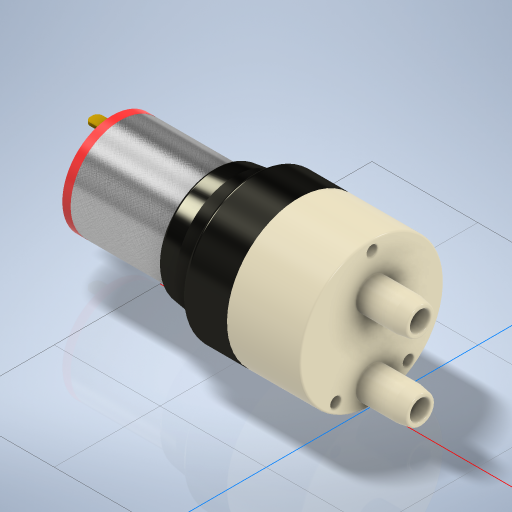
# Autodesk Inventor part: pump
Saved by Autodesk Inventor 2024 (Build 280153000, 153)
## iProperties
Created: 2023-05-18
Part Number: pump
Material: Generic
Document SubType Name: Modeling
Designer: jeff7
Density: 1 g/cm^3
Appearance: Default
Author: jeff7
Autodesk Inventor part; units mm, degrees
sketch "Sketch1" plane through (0, 0, 0) normal (1, 0, 0) x (0, 1, 0)
  circle A0 centre (0, 0) radius 17.25
  dimension "d0" = 34.5
  constraints: 2 coincident, 1 centre point
  measures "d0" diameter of A0
extrude "Extrusion1" add sketch "Sketch1" against normal blind 28.4
sketch "Sketch2" plane through (-28.4, 0, 0) normal (-1, 0, 0) x (0, 0, 1)
  circle A0 centre (0, 0) radius 14.1
  dimension "d3" = 28.2
  constraints: 1 centre point, 1 coincident
  measures "d3" diameter of A0
extrude "Extrusion2" add sketch "Sketch2" along normal blind 9.5
sketch "Sketch3" plane through (-37.9, 0, 0) normal (-1, 0, 0) x (0, 0, 1)
  circle A0 centre (0, 0) radius 17.25 projected
  circle A1 centre (0, 0) radius 11.95
  dimension "d6" = 23.9
  constraints: 1 centre point, 1 coincident
  measures "d6" diameter of A1
extrude "Extrusion3" add sketch "Sketch3" along normal blind 24.4 contours A1
sketch "Sketch5" plane through (0, 0, 0) normal (1, 0, 0) x (0, 0, -1)
  circle A0 centre (0, -12.35) radius 3.85
  circle A1 centre (0, 6.1) radius 3.85
  circle A2 centre (0, -12.35) radius 2.35
  circle A3 centre (0, 6.1) radius 2.35
  circle A4 centre (0, 0) radius 17.25 projected
  dimension "d9" = 7.7
  dimension "d10" = 7.7
  dimension "d11" = 4.7
  dimension "d12" = 4.7
  dimension "d13" = 1.05
  dimension "d14" = 15
  constraints: 4 centre point, 2 coincident, 2 vertical alignment
  measures "d9" diameter of A0
  measures "d10" diameter of A1
  measures "d11" diameter of A2
  measures "d12" diameter of A3
extrude "Extrusion4" add sketch "Sketch5" along normal blind 11.7 contours A0 | A1
sketch "Sketch6" plane through (0, 0, 0) normal (1, 0, 0) x (0, 0, -1)
  circle A0 centre (0, 14.95) radius 1.3
  circle A1 centre (8.7, -12.1578) radius 1.3
  circle A2 centre (-8.7, -12.1578) radius 1.3
  circle A3 centre (0, 0) radius 17.25 projected
  dimension "d17" = 2.6
  dimension "d18" = 2.6
  dimension "d19" = 2.6
  dimension "d20" = 1
  dimension "d21" = 17.4
  dimension "d22" = 1
  dimension "d23" = 1
  constraints: 3 centre point, 1 horizontal alignment, 1 vertical alignment
  measures "d17" diameter of A0
  measures "d18" diameter of A2
  measures "d19" diameter of A1
  measures "d21" distance of A1.centre A2.centre
extrude "Extrusion5" cut sketch "Sketch6" against normal blind 10 contours A0 | A1 | A2
ref_plane "Work Plane1" through (-17.5, 0, 0) normal (1, 0, 0) x (0, 0, -1)
split body "Split" result two bodies by plane through (-17.5, 0, 0) normal (1, 0, 0) first body at (-11.6667, 16.6957, -1.3478)
ref_plane "Work Plane2" through (-37.9, 0, 0) normal (1, 0, 0) x (0, 0, -1)
split body "Split4" result two bodies by plane through (-37.9, 0, 0) normal (1, 0, 0) bodies 3 first body at (-24.7667, 16.6957, -1.3478)
ref_plane "Work Plane3" through (-60.3, 0, 0) normal (-1, 0, 0) x (0, 0, 1)
split body "Split5" result two bodies by plane through (-60.3, 0, 0) normal (-1, 0, 0) bodies 5 first body at (-60.8, -1.8511, -3.5271)
sketch "Sketch8" plane through (-62.3, 0, 0) normal (-1, 0, 0) x (0, 0, 1)
  line L0 (-1.5, 9.3) -> (1.5, 9.3)
  line L1 (1.5, 9.3) -> (1.5, 8.6)
  line L2 (1.5, 8.6) -> (-1.5, 8.6)
  line L3 (-1.5, 8.6) -> (-1.5, 9.3)
  line L4 (-1.5, -8.6) -> (1.5, -8.6)
  line L5 (1.5, -8.6) -> (1.5, -9.3)
  line L6 (1.5, -9.3) -> (-1.5, -9.3)
  line L7 (-1.5, -9.3) -> (-1.5, -8.6)
  point P0 (0, 0)
  point P1 (0, 8.6)
  dimension "d29" = 3
  dimension "d30" = 0.7
  dimension "d31" = 0.7
  dimension "d32" = 8.6
  dimension "d33" = 8.6
  constraints: 16 end point, 4 parallel, 2 horizontal, 2 perpendicular, 2 point on line, 1 midpoint, 1 vertical alignment
  measures "d29" distance of L0.start L0.end
  measures "d30" distance between parallel lines of L6 L4
  measures "d31" distance between parallel lines of L0 L2
  measures "d32" distance from line of point (0, 0) L2
  measures "d33" distance from line of point (0, 0) L4
extrude "Extrusion6" add sketch "Sketch8" along normal blind 5 bodies 6
chamfer "Chamfer3" distance 0.7 distance2 5 1 edges at (-37.9, 0, -14.1) measured on face at (-37.9, 0, -13.6)
fillet "Fillet1" radius 1 3 edges at (-28.4, 0, -14.1) (-28.4, -17.25, 0) (-37.9, 0, -13.4)
ref_plane "Work Plane4" through (-62.3, 0, 0) normal (-1, 0, 0) x (0, 0, 1)
split body "Split6" result two bodies by plane through (-62.3, 0, 0) normal (-1, 0, 0) bodies 6 first body at (-65.6333, -9.1, 0.5) (-65.6333, 8.8, 0.5)
fillet "Fillet2" radius 1.2 4 edges at (-67.3, 8.95, 1.5) (-67.3, 8.95, -1.5) (-67.3, -8.95, 1.5) (-67.3, -8.95, -1.5)
chamfer "Chamfer1" distance 0.5 distance2 3 1 edges at (11.7, -12.35, 3.85) measured on face at (11.7, -12.35, 3.35)
chamfer "Chamfer2" distance 0.5 distance2 3 1 edges at (11.7, 6.1, 3.85) measured on face at (11.7, 6.1, 3.35)
fillet "Fillet3" radius 0.4 5 edges at (11.7, 6.1, 2.35) (11.7, 6.1, 3.35) (11.7, -12.35, 2.35) (11.7, -12.35, 3.35) (0, -17.25, 0)
equation "\"wall_thick\" = 3"
body "Solid1"
body "Solid2"
body "Solid4"
body "Solid7"
body "Solid8"
body "Solid9"
